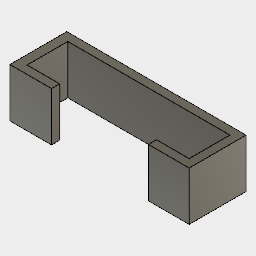
psu-holder (Autodesk Fusion 360 design; units mm, degrees)
Autodesk Fusion 360 part; units mm, degrees
sketch "Sketch1" plane through (0, 0, 0) normal (0, 0, 1) x (1, 0, 0)
sketch "Sketch2" plane through (0, 0, 0) normal (0, 0, 1) x (1, 0, 0)
  line L0 (14.5953, 39.9307) -> (124.5953, 39.9307)
  line L1 (124.5953, 39.9307) -> (124.5953, 34.9307)
  line L2 (124.5953, 34.9307) -> (14.5953, 34.9307)
  line L3 (14.5953, 34.9307) -> (14.5953, 39.9307)
  line L4 (14.5953, 34.9307) -> (20.2023, 34.9307)
  line L5 (20.2023, 34.9307) -> (20.2023, 4.9307)
  line L6 (20.2023, 4.9307) -> (14.5953, 4.9307)
  line L7 (14.5953, 4.9307) -> (14.5953, 34.9307)
  line L8 (124.5953, 34.9307) -> (124.5953, 4.9307)
  line L9 (124.5953, 4.9307) -> (119.5953, 4.9307)
  line L10 (119.5953, 4.9307) -> (119.5953, 34.9307)
  line L11 (20.2023, 9.9307) -> (40.2023, 9.9307)
  line L12 (40.2023, 9.9307) -> (40.2023, 4.9307)
  line L13 (40.2023, 4.9307) -> (20.2023, 4.9307)
  line L14 (20.2023, 4.9307) -> (20.2023, 9.9307)
  line L15 (99.5953, 9.9307) -> (119.5953, 9.9307)
  line L16 (119.5953, 9.9307) -> (119.5953, 4.9307)
  line L17 (119.5953, 4.9307) -> (99.5953, 4.9307)
  line L18 (99.5953, 4.9307) -> (99.5953, 9.9307)
  dimension "d1" = 110
  dimension "d2" = 5
  dimension "d3" = 30
  dimension "d4" = 5
  dimension "d5" = 30
  dimension "d6" = 20
  dimension "d7" = 5
  dimension "d8" = 20
  dimension "d9" = 5
  measures "d1" distance of L0.start L0.end
  measures "d2" distance of L0.start L2.end
  measures "d3" distance of L2.end L6.end
  measures "d4" distance of L10.end L1.end
  measures "d5" distance of L10.end L9.end
  measures "d6" distance of L11.start L11.end
  measures "d7" distance of L11.start L5.end
  measures "d8" distance of L15.start L15.end
  measures "d9" distance of L15.start L17.end
extrude "Extrude1" add sketch "Sketch2" along normal blind 30
